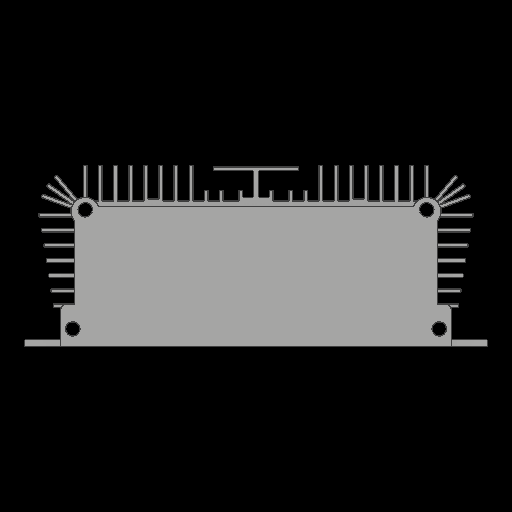
# Autodesk Inventor part: Daygreen-A2D12C100-Converter
Saved by Autodesk Inventor 2025.2 (Build 292293000, 293)
## iProperties
Created: 2025-11-13
Part Number: Daygreen-A2D12C100-Converter
Material: Generic
Document SubType Name: Modeling
Designer: valer
Density: 1 g/cm^3
Appearance: Default
Author: valer
Autodesk Inventor part; units mm, degrees
ref_plane "YZ Plane" through (0, 0, 0) normal (1, 0, 0) x (0, 1, 0)
ref_plane "XZ Plane" through (0, 0, 0) normal (0, 1, 0) x (-1, 0, 0)
sketch "Base" plane through (0, 0, 0) normal (0, 0, 1) x (1, 0, 0)
  line L0 (-65, -111.5) -> (65, -111.5)
  line L1 (65, -111.5) -> (65, 111.5)
  line L2 (65, 111.5) -> (-65, 111.5)
  line L3 (-65, 111.5) -> (-65, -111.5)
  line L4 (-65, -111.5) -> (65, 111.5) construction
  line L5 (65, -111.5) -> (-65, 111.5) construction
  line L6 (-91, 0) -> (91, 0) construction
  line L7 (0, -156.1) -> (0, 156.1) construction
  circle A0 centre (-59.5, 75.5) radius 2.5
  line L8 (-59.5, 78) -> (-65, 78)
  line L9 (-59.5, 73) -> (-65, 73)
  line L10 (-57, 75.5) -> (-65, 75.5) construction
  circle A1 centre (-59.5, 0) radius 2.5
  line L11 (-59.5, 2.5) -> (-65, 2.5)
  line L12 (-59.5, -2.5) -> (-65, -2.5)
  circle A2 centre (-59.5, -75.5) radius 2.5
  line L13 (-59.5, -78) -> (-65, -78)
  line L14 (-59.5, -73) -> (-65, -73)
  circle A3 centre (59.5, 75.5) radius 2.5
  line L15 (59.5, 78) -> (65, 78)
  line L16 (59.5, 73) -> (65, 73)
  circle A4 centre (59.5, 0) radius 2.5
  line L17 (59.5, 2.5) -> (65, 2.5)
  line L18 (59.5, -2.5) -> (65, -2.5)
  line L19 (59.5, -78) -> (65, -78)
  line L20 (59.5, -73) -> (65, -73)
  circle A5 centre (59.5, -75.5) radius 2.5
  point P0 (0, 0)
  dimension "d0" = 130
  dimension "d1" = 223
  dimension "d4" = 5
  dimension "d5" = 8
  dimension "d6" = 36
  constraints: 38 end point, 20 symmetric about line, 13 point on circle, 7 point on line, 6 centre point, 6 perpendicular, 4 tangent, 3 parallel, 2 midpoint, 1 equal radius, 1 horizontal, 4 other
  measures "d0" distance of L1.end L2.end
  measures "d1" distance of L0.end L1.end
  measures "d4" diameter of A0
  measures "d5" distance of L10.start L10.end
  measures "d6" distance between parallel lines of L10 L2
extrude "BaseFeature" add sketch "Base" along normal blind 2 contours L3 L13 A2 L14 L12 A1 L11 L9 A0 L8 L2 L1 L15 A3 L16 L17 A4 L18 L20 A5 L19 L0
sketch "BaseIndent" plane through (0, 0, 0) normal (0, 0, 1) x (1, 0, 0)
  line L0 (65, 111.5) -> (-65, 111.5) projected
  line L1 (-65, -111.5) -> (65, -111.5) projected
  line L2 (47.62, 111.5) -> (-47.62, 111.5)
  line L3 (-47.62, 111.5) -> (-47.62, -111.5)
  line L4 (-47.62, -111.5) -> (47.62, -111.5)
  line L5 (47.62, -111.5) -> (47.62, 111.5)
  line L6 (-65, 111.5) -> (-65, 78) projected
  line L7 (65, 78) -> (65, 111.5) projected
  point P0 (0, 0)
  point P1 (47.62, -111.5)
  point P2 (-47.62, 111.5)
  dimension "d7" = 17.38
  dimension "d8" = 17.38
  constraints: 8 end point, 2 parallel, 2 point on line, 1 horizontal, 1 perpendicular
  measures "d7" distance between parallel lines of L6 L3
  measures "d8" distance between parallel lines of L7 L5
extrude "BaseIndentFeature" cut sketch "BaseIndent" along normal blind 0.5
sketch "Wall" plane through (-65, -111.5, 2) normal (0, -1, 0) x (1, 0, 0)
  line L0 (0, -2) -> (17.38, -2) projected
  line L1 (10, -2) -> (120, -2)
  line L2 (120, -2) -> (120, 10)
  line L3 (120, 10) -> (10, 10)
  line L4 (10, 10) -> (10, -2)
  line L5 (14, 10) -> (116, 10)
  line L6 (116, 10) -> (116, 37.5)
  line L7 (116, 37.5) -> (14, 37.5)
  line L8 (14, 37.5) -> (14, 10)
  circle A0 centre (17, 36) radius 4
  line L9 (65, -10.5958) -> (65, 49.5748) construction
  line L10 (0, -2) -> (0, 0) projected
  circle A1 centre (113, 36) radius 4
  circle A2 centre (13.5, 3) radius 2
  line L11 (0, 0) -> (130, 0) projected
  circle A3 centre (17, 36.5) radius 2
  circle A4 centre (116.5, 3) radius 2
  circle A5 centre (113, 36.5) radius 2
  point P0 (65, -2)
  point P1 (65, 37.5)
  point P2 (65, 10)
  point P3 (20.7081, 37.5)
  point P4 (14, 33.3542)
  point P5 (116, 10)
  point P6 (116, 33.3542)
  point P7 (109.2919, 37.5)
  dimension "d11" = 12
  dimension "d12" = 39.5
  dimension "d13" = 102
  dimension "d14" = 10
  dimension "d18" = 8
  dimension "d19" = 48
  dimension "d20" = 1.5
  dimension "d21" = 4
  dimension "d24" = 3.5
  dimension "d25" = 5
  dimension "d27" = 3
  dimension "d28" = 1
  dimension "d61" = 4
  constraints: 16 end point, 6 centre point, 4 parallel, 3 midpoint, 3 point on line, 3 symmetric about line, 2 horizontal, 2 perpendicular, 3 other
  measures "d11" distance between parallel lines of L0 L3
  measures "d12" distance between parallel lines of L0 L7
  measures "d13" distance of L7.end L6.end
  measures "d14" distance between parallel lines of L10 L4
  measures "d18" diameter of A0
  measures "d19" distance from line of L9 A0.centre
  measures "d20" distance from line of L7 A0.centre
  measures "d21" diameter of A2
  measures "d24" distance from line of L4 A2.centre
  measures "d25" distance from line of L0 A2.centre
  measures "d27" distance from line of L8 A3.centre
  measures "d28" distance from line of L7 A3.centre
  measures "d61" diameter of A5
extrude "WallFeature" add sketch "Wall" along normal blind 1.6 contours L4 L11 L2 L1 L0 | L4 L3 L2 L11 | L8 A0 L7 A1 L6 L3 | A0 L7 A3 L8 | L8 L7 A3 A0 | A1 L7 A5 L6 | L6 L7 A5 A1
mirror "WallMirrorFeature" about plane through (0, 0, 0) normal (0, 1, 0) of "WallFeature"
fillet "WallFilletsFeature" radius 2 4 edges at (-55, -112.3, 12) (55, -112.3, 12) (-55, 112.3, 12) (55, 112.3, 12)
sketch "Heatsink" plane through (-65, -111.5, 2) normal (0, 1, 0) x (1, 0, 0)
  arc A0 (14, -33.3542) -> (20.7081, -37.5) centre (17, -36) ccw projected
  line L0 (19.6458, -39) -> (20.75, -39)
  line L1 (20.75, -39) -> (20.75, -49)
  line L2 (20.75, -49) -> (21.75, -49)
  line L3 (21.75, -49) -> (21.75, -39)
  line L4 (21.75, -39) -> (25, -39)
  line L5 (25, -39) -> (25, -49)
  line L6 (25, -49) -> (26, -49)
  line L7 (26, -49) -> (26, -39)
  line L8 (26, -39) -> (29.25, -39)
  line L9 (29.25, -39) -> (29.25, -49)
  line L10 (29.25, -49) -> (30.25, -49)
  line L11 (30.25, -49) -> (30.25, -39)
  line L12 (30.25, -39) -> (33.5, -39)
  line L13 (33.5, -39) -> (33.5, -49)
  line L14 (33.5, -49) -> (34.5, -49)
  line L15 (34.5, -49) -> (34.5, -39.5)
  line L16 (34.5, -39.5) -> (37.75, -39.5)
  line L17 (37.75, -39.5) -> (37.75, -49)
  line L18 (37.75, -49) -> (38.75, -49)
  line L19 (38.75, -49) -> (38.75, -39)
  line L20 (38.75, -39) -> (42, -39)
  line L21 (42, -39) -> (42, -49)
  line L22 (42, -49) -> (43, -49)
  line L23 (43, -49) -> (43, -39)
  line L24 (43, -39) -> (46.25, -39)
  line L25 (46.25, -39) -> (46.25, -49)
  line L26 (46.25, -49) -> (47.25, -49)
  line L27 (47.25, -49) -> (47.25, -39)
  line L28 (47.25, -39) -> (50.5, -39)
  line L29 (50.5, -39) -> (50.5, -42)
  line L30 (50.5, -42) -> (51.5, -42)
  line L31 (51.5, -42) -> (51.5, -39)
  line L32 (51.5, -39) -> (54.75, -39)
  line L33 (54.75, -39) -> (54.75, -42)
  line L34 (54.75, -42) -> (55.75, -42)
  line L35 (55.75, -42) -> (55.75, -39)
  line L36 (55.75, -39) -> (60.25, -39)
  line L37 (60.25, -39) -> (60.25, -42)
  line L38 (60.25, -42) -> (61.25, -42)
  line L39 (61.25, -42) -> (61.25, -40)
  line L40 (61.25, -40) -> (64.25, -40)
  line L41 (64.25, -40) -> (64.25, -47.5)
  line L42 (64.25, -47.5) -> (53, -47.5)
  line L43 (53, -47.5) -> (53, -48.5)
  line L44 (53, -48.5) -> (65, -48.5)
  line L45 (65, -48.5) -> (65, -37.5)
  line L46 (109.2919, -37.5) -> (20.7081, -37.5) projected
  line L47 (20.75, -39) -> (19.6458, -39)
  line L48 (17.5, -49) -> (17.5, -39.9686)
  line L49 (17.5, -49) -> (16.5, -49)
  line L50 (16.5, -49) -> (16.5, -39.9686)
  line L51 (14.832, -39.3615) -> (9.0268, -46.28)
  line L52 (9.0268, -46.28) -> (8.2607, -45.6372)
  line L53 (8.2607, -45.6372) -> (14.066, -38.7188)
  line L54 (14.0359, -38.6859) -> (6.6378, -43.8661)
  line L55 (6.6378, -43.8661) -> (6.0642, -43.0469)
  line L56 (6.0642, -43.0469) -> (13.4623, -37.8667)
  line L57 (13.0997, -36.8875) -> (4.613, -39.9764)
  line L58 (4.613, -39.9764) -> (4.955, -40.9161)
  line L59 (4.955, -40.9161) -> (13.4417, -37.8272)
  line L60 (4.0385, -35.5) -> (13.0314, -35.5)
  line L61 (4.0385, -35.5) -> (4.0385, -34.5)
  line L62 (4.0385, -34.5) -> (13.2919, -34.5)
  line L63 (14, -33.3542) -> (14, -10) projected
  line L64 (14, -31.25) -> (4.712, -31.25)
  line L65 (4.712, -31.25) -> (4.712, -30.25)
  line L66 (4.712, -30.25) -> (14, -30.25)
  line L67 (14, -27) -> (5.3854, -27)
  line L68 (5.3854, -27) -> (5.3854, -26)
  line L69 (5.3854, -26) -> (14, -26)
  line L70 (14, -22.75) -> (6.0589, -22.75)
  line L71 (6.0589, -22.75) -> (6.0589, -21.75)
  line L72 (6.0589, -21.75) -> (14, -21.75)
  line L73 (14, -18.5) -> (6.7323, -18.5)
  line L74 (6.7323, -18.5) -> (6.7323, -17.5)
  line L75 (6.7323, -17.5) -> (14, -17.5)
  line L76 (14, -14.25) -> (7.4058, -14.25)
  line L77 (7.4058, -14.25) -> (7.4058, -13.25)
  line L78 (7.4058, -13.25) -> (14, -13.25)
  line L79 (14, -10) -> (8, -10)
  line L80 (8, -10) -> (8, -9)
  line L81 (8, -9) -> (10.2679, -9)
  arc A1 (10, -8) -> (12, -10) centre (12, -8) ccw projected
  line L82 (6.351, -43.4565) -> (17, -36) construction
  line L83 (4.784, -40.4463) -> (17, -36) construction
  line L84 (8.6438, -45.9586) -> (17, -36) construction
  circle A2 centre (17, -36) radius 13 construction
  line L85 (4.0385, -35) -> (8, -10) construction
  line L86 (10, -8) -> (10, 2) projected
  line L87 (65, 12.2) -> (65, -59.2) construction
  line L88 (65, -37.5) -> (65, 2)
  line L89 (10, 2) -> (120, 2) projected
  line L90 (14, -10) -> (12, -10) projected
  arc A3 (118, -10) -> (120, -8) centre (118, -8) ccw projected
  line L91 (118, -10) -> (116, -10) projected
  line L92 (116, -10) -> (116, -33.3542) projected
  arc A4 (109.2919, -37.5) -> (116, -33.3542) centre (113, -36) ccw projected
  line L93 (109.2919, -37.5) -> (20.7081, -37.5) projected
  arc A5 (14, -33.3542) -> (20.7081, -37.5) centre (17, -36) ccw projected
  line L94 (14, -33.3542) -> (14, -10) projected
  line L95 (14, -10) -> (12, -10) projected
  arc A6 (10, -8) -> (12, -10) centre (12, -8) ccw projected
  line L96 (10, -8) -> (10, 2) projected
  line L97 (10, 2) -> (120, 2) projected
  line L98 (120, 2) -> (120, -8) projected
  circle A7 centre (17, -36.5) radius 2 projected
  circle A8 centre (116.5, -3) radius 2 projected
  circle A9 centre (13.5, -3) radius 2 projected
  circle A10 centre (113, -36.5) radius 2 projected
  point P0 (48.875, -39)
  point P1 (51, -42)
  point P2 (7.4058, -13.75)
  point P3 (6.7323, -18)
  point P4 (6.0589, -22.25)
  point P5 (5.3854, -26.5)
  point P6 (4.712, -30.75)
  dimension "d30" = 12
  dimension "d31" = 11
  dimension "d32" = 1
  dimension "d33" = 1.5
  dimension "d34" = 3.25
  dimension "d35" = 2
  dimension "d36" = 2.5
  dimension "d37" = 10
  dimension "d38" = 3
  dimension "d39" = 4.5
  dimension "d40" = 0.75
  dimension "d41" = 125
  dimension "d42" = 15
  dimension "d43" = 15
  dimension "d44" = 3.25
  dimension "d45" = 3.25
  dimension "d46" = 3.25
  dimension "d47" = 3.25
  dimension "d48" = 3.25
  dimension "d49" = 3.25
  dimension "d50" = 20
  dimension "d51" = 40
  dimension "d52" = 2
  dimension "d53" = 3.25
  dimension "d54" = 3
  constraints: 170 end point, 45 perpendicular, 29 equal length, 17 collinear, 14 horizontal, 12 midpoint, 9 point on line, 8 parallel, 5 point on circle, 1 centre point, 1 coincident, 1 vertical, 23 other
  measures "d30" distance of L43.end L44.end
  measures "d31" distance of L44.end L45.end
  measures "d32" distance between parallel lines of L3 L1
  measures "d33" distance between parallel lines of L46 L4
  measures "d34" distance between parallel lines of L5 L3
  measures "d35" distance between parallel lines of L46 L16
  measures "d36" distance between parallel lines of L46 L40
  measures "d37" distance of L0.end L1.end
  measures "d38" vertical distance of point (48.875, -39) point (51, -42)
  measures "d39" distance of L35.end L36.end
  measures "d40" distance between parallel lines of L45 L41
  measures "d42" angle of L53 L54
  measures "d43" angle of L59 L56
  measures "d44" distance between parallel lines of L79 L78
  measures "d45" distance between parallel lines of L76 L75
  measures "d46" distance between parallel lines of L73 L72
  measures "d47" distance between parallel lines of L70 L69
  measures "d48" distance between parallel lines of L67 L66
  measures "d49" distance between parallel lines of L64 L62
  measures "d50" angle of L60 L57
  measures "d51" angle of L50 L51
  measures "d52" distance from line of L86 L80.end
  measures "d53" distance between parallel lines of L48 L1
  measures "d54" distance of L39.end L40.end
extrude "HeatSinkFeature" add sketch "Heatsink" along normal up to surface (223 mm away) contours L63 L79 A1 L86 L89 L88 L46 A0 | A0 L60 L61 L62 | L64 L65 L66 L63 | A0 L59 L58 L57 | L67 L68 L69 L63 | A0 L54 L55 L56 | L70 L71 L72 L63 | A0 L51 L52 L53 | L73 L74 L75 L63 | A0 L48 L49 L50 | L76 L77 L78 L63 | A0 L46 L45 L44 L43 L42 L41 L40 L39 L38 L37 L36 L35 L34 L33 L32 L31 L30 L29 L28 L27 L26 L25 L24 L23 L22 L21 L20 L19 L18 L17 L16 L15 L14 L13 L12 L11 L10 L9 L8 L7 L6 L5 L4 L3 L2 L1 L0 | L79 L80 L81 A1
mirror "HeatSinkMirrorFeature" about plane through (0, 0, 0) normal (1, 0, 0) of "HeatSinkFeature"
sketch "Terminal" plane through (-55, 113.1, 0) normal (0, 1, 0) x (1, 0, 0)
  line L0 (94.25, -26) -> (15.75, -26)
  line L1 (15.75, -26) -> (15.75, -13)
  line L2 (15.75, -13) -> (94.25, -13)
  line L3 (94.25, -13) -> (94.25, -26)
  line L4 (55, 10.2) -> (55, -61.2) construction
  line L5 (99.2919, -39.5) -> (10.7081, -39.5) projected
  line L6 (55, -39.5) -> (55, 0) construction
  line L7 (0, 0) -> (110, 0) projected
  point P0 (55, 0)
  point P1 (55, -26)
  dimension "d57" = 78.5
  dimension "d58" = 13
  dimension "d59" = 13
  dimension "d60" = 13.5
  constraints: 10 end point, 3 midpoint, 2 parallel, 2 point on line, 1 horizontal, 1 perpendicular
  measures "d57" distance of L0.start L0.end
  measures "d58" distance of L2.end L0.start
  measures "d59" distance between parallel lines of L7 L2
  measures "d60" distance between parallel lines of L5 L0
extrude "TerminalFeature" add sketch "Terminal" along normal blind 11.7
sketch "TerminalCells" plane through (-39.25, 113.1, 26) normal (0, 0, 1) x (1, 0, 0)
  line L0 (78.5, 11.7) -> (0, 11.7) projected
  line L1 (2.5, 11.7) -> (14.2, 11.7)
  line L2 (14.2, 11.7) -> (14.2, 0)
  line L3 (14.2, 0) -> (2.5, 0)
  line L4 (2.5, 0) -> (2.5, 11.7)
  line L5 (16.7, 11.7) -> (28.4, 11.7)
  line L6 (28.4, 11.7) -> (28.4, 0)
  line L7 (28.4, 0) -> (16.7, 0)
  line L8 (16.7, 0) -> (16.7, 11.7)
  line L9 (76, 11.7) -> (64.3, 11.7)
  line L10 (64.3, 11.7) -> (64.3, 0)
  line L11 (64.3, 0) -> (76, 0)
  line L12 (76, 0) -> (76, 11.7)
  line L13 (61.8, 11.7) -> (53.5, 11.7)
  line L14 (53.5, 11.7) -> (53.5, 0)
  line L15 (53.5, 0) -> (61.8, 0)
  line L16 (61.8, 0) -> (61.8, 11.7)
  line L17 (51, 11.7) -> (39.3, 11.7)
  line L18 (39.3, 11.7) -> (39.3, 0)
  line L19 (39.3, 0) -> (51, 0)
  line L20 (51, 0) -> (51, 11.7)
  line L21 (83.5419, 0) -> (-5.0419, 0) projected
  line L22 (0, 0) -> (0, 11.7) projected
  line L23 (78.5, 0) -> (78.5, 11.7) projected
  point P0 (39.25, -113.1)
  point P1 (51, 11.7)
  point P2 (39.3, 11.7)
  dimension "d64" = 11.7
  dimension "d65" = 2.5
  dimension "d66" = 2.5
  dimension "d67" = 2.5
  dimension "d68" = 2.5
  dimension "d69" = 2.5
  dimension "d70" = 8.3
  constraints: 40 end point, 10 parallel, 8 point on line, 5 collinear, 5 horizontal, 5 perpendicular
  measures "d64" distance between parallel lines of L12 L10
  measures "d65" distance between parallel lines of L4 L22
  measures "d66" distance between parallel lines of L8 L2
  measures "d67" distance between parallel lines of L23 L12
  measures "d68" distance between parallel lines of L16 L10
  measures "d69" distance between parallel lines of L14 L20
  measures "d70" distance between parallel lines of L16 L14
extrude "TerminalCellsFeature" cut sketch "TerminalCells" against normal blind 6 contours L12 L11 L10 L0 | L16 L15 L14 L0 | L20 L19 L18 L0 | L6 L7 L8 L0 | L2 L3 L4 L0
sketch "TerminalBreak" plane through (-10.85, 113.1, 26) normal (0, 0, 1) x (1, 0, 0)
  line L0 (10.9, 0) -> (10.9, 11.7) projected
  line L1 (0, 11.7) -> (10.9, 11.7) projected
  line L2 (0, 11.7) -> (0, 0) projected
  line L3 (10.9, 0) -> (0, 0) projected
  line L4 (2.5, 0) -> (2.5, 11.7)
  line L5 (8.4, 0) -> (8.4, 11.7)
  point P0 (10.85, -113.1)
  dimension "d73" = 2.5
  dimension "d74" = 2.5
  constraints: 4 end point, 4 point on line, 2 perpendicular
  measures "d73" distance between parallel lines of L2 L4
  measures "d74" distance between parallel lines of L0 L5
extrude "TerminalBreakFeature" cut sketch "TerminalBreak" against normal through all contours L3 L4 L1 L5
sketch "TerminalChannels" plane through (-55, 124.8, 0) normal (0, 1, 0) x (1, 0, 0)
  line L0 (46.65, -26) -> (46.65, -13) projected
  line L1 (46.65, -13) -> (15.75, -13) projected
  line L2 (15.75, -13) -> (15.75, -26) projected
  line L3 (15.75, -26) -> (18.25, -26) projected
  line L4 (18.25, -26) -> (18.25, -20) projected
  line L5 (18.25, -20) -> (29.95, -20) projected
  line L6 (29.95, -20) -> (29.95, -26) projected
  line L7 (29.95, -26) -> (32.45, -26) projected
  line L8 (32.45, -26) -> (32.45, -20) projected
  line L9 (32.45, -20) -> (44.15, -20) projected
  line L10 (44.15, -20) -> (44.15, -26) projected
  line L11 (44.15, -26) -> (46.65, -26) projected
  line L12 (52.55, -13) -> (52.55, -26) projected
  line L13 (52.55, -26) -> (55.05, -26) projected
  line L14 (55.05, -26) -> (55.05, -20) projected
  line L15 (55.05, -20) -> (66.75, -20) projected
  line L16 (66.75, -20) -> (66.75, -26) projected
  line L17 (66.75, -26) -> (69.25, -26) projected
  line L18 (69.25, -26) -> (69.25, -20) projected
  line L19 (69.25, -20) -> (77.55, -20) projected
  line L20 (77.55, -20) -> (77.55, -26) projected
  line L21 (77.55, -26) -> (80.05, -26) projected
  line L22 (80.05, -26) -> (80.05, -20) projected
  line L23 (80.05, -20) -> (91.75, -20) projected
  line L24 (91.75, -20) -> (91.75, -26) projected
  line L25 (91.75, -26) -> (94.25, -26) projected
  line L26 (94.25, -26) -> (94.25, -13) projected
  line L27 (94.25, -13) -> (52.55, -13) projected
  line L28 (31.2, -26) -> (31.2, -13)
  line L29 (29.95, -20) -> (18.25, -20) projected
  line L30 (28.35, -20) -> (28.1, -15)
  line L31 (28.1, -15) -> (20.1, -15)
  line L32 (20.1, -15) -> (19.85, -20)
  line L33 (24.1, -15) -> (24.1, -20) construction
  line L34 (34.05, -20) -> (34.3, -15)
  line L35 (34.3, -15) -> (42.3, -15)
  line L36 (42.3, -15) -> (42.55, -20)
  line L37 (73.4, -20) -> (73.4, -13) construction
  line L38 (65.15, -20) -> (64.9, -15)
  line L39 (64.9, -15) -> (56.9, -15)
  line L40 (56.9, -15) -> (56.65, -20)
  line L41 (66.75, -20) -> (55.05, -20) projected
  line L42 (60.9, -20) -> (60.9, -15) construction
  line L43 (81.65, -20) -> (81.9, -15)
  line L44 (81.9, -15) -> (89.9, -15)
  line L45 (89.9, -15) -> (90.15, -20)
  point P0 (55, 0)
  point P1 (19.85, -20)
  point P2 (42.55, -20)
  dimension "d77" = 8.5
  dimension "d78" = 8
  dimension "d79" = 2
  dimension "d80" = 8.5
  constraints: 32 end point, 8 midpoint, 8 symmetric about line, 4 point on line, 3 equal length, 2 perpendicular, 1 collinear, 1 horizontal, 1 parallel
  measures "d77" distance of L32.end L30.start
  measures "d78" distance of L30.end L31.end
  measures "d79" distance between parallel lines of L1 L31
  measures "d80" distance of L40.end L38.start
extrude "TerminalChannelsFeature" cut sketch "TerminalChannels" against normal up to surface (11.7 mm away) contours L9 L34 L35 L36 | L5 L32 L31 L30 | L40 L39 L38 L15 | L23 L43 L44 L45
ref_plane "TerminalPlatePlane" through (-55, 125.05, 0) normal (0, 1, 0) x (1, 0, 0)
sketch "TerminalPlates" plane through (-55, 125.05, 0) normal (0, 1, 0) x (1, 0, 0)
  line L0 (29.95, -26) -> (29.95, -20) projected
  line L1 (18.25, -26) -> (18.25, -20) projected
  line L2 (29.95, -20) -> (18.25, -20)
  line L3 (18.25, -20) -> (18.25, -21)
  line L4 (18.25, -21) -> (29.95, -21)
  line L5 (29.95, -21) -> (29.95, -20)
  line L6 (44.15, -26) -> (44.15, -20) projected
  line L7 (32.45, -26) -> (32.45, -20) projected
  line L8 (44.15, -20) -> (32.45, -20)
  line L9 (32.45, -20) -> (32.45, -21)
  line L10 (32.45, -21) -> (44.15, -21)
  line L11 (44.15, -21) -> (44.15, -20)
  line L12 (66.75, -26) -> (66.75, -20) projected
  line L13 (55.05, -26) -> (55.05, -20) projected
  line L14 (66.75, -20) -> (55.05, -20)
  line L15 (55.05, -20) -> (55.05, -21)
  line L16 (55.05, -21) -> (66.75, -21)
  line L17 (66.75, -21) -> (66.75, -20)
  line L18 (91.75, -26) -> (91.75, -20) projected
  line L19 (80.05, -26) -> (80.05, -20) projected
  line L20 (91.75, -20) -> (80.05, -20)
  line L21 (80.05, -20) -> (80.05, -21)
  line L22 (80.05, -21) -> (91.75, -21)
  line L23 (91.75, -21) -> (91.75, -20)
  point P0 (55, 0)
  point P1 (18.25, -20)
  point P2 (29.95, -21)
  point P3 (32.45, -20)
  point P4 (91.75, -21)
  dimension "d84" = 1
  constraints: 32 end point, 8 parallel, 4 horizontal, 4 perpendicular, 4 point on line, 3 collinear
  measures "d84" distance from line of L1.end L4
extrude "TerminalPlatesFeature" add sketch "TerminalPlates" against normal up to surface (11.95 mm away)
sketch "TerminalBoltRings" plane through (-36.75, 125.05, 21) normal (0, 0, 1) x (1, 0, 0)
  line L0 (11.7, -11.95) -> (0, -11.95) projected
  line L1 (11.7, -0.25) -> (11.7, -11.95) projected
  line L2 (11.7, 0) -> (11.7, -0.25) projected
  line L3 (0, 0) -> (11.7, 0) projected
  line L4 (0, 0) -> (0, -0.25) projected
  line L5 (0, -11.95) -> (0, -0.25) projected
  line L6 (25.9, -11.95) -> (14.2, -11.95) projected
  line L7 (25.9, -0.25) -> (25.9, -11.95) projected
  line L8 (25.9, 0) -> (25.9, -0.25) projected
  line L9 (14.2, 0) -> (25.9, 0) projected
  line L10 (14.2, 0) -> (14.2, -0.25) projected
  line L11 (14.2, -11.95) -> (14.2, -0.25) projected
  line L12 (48.5, -11.95) -> (36.8, -11.95) projected
  line L13 (48.5, -0.25) -> (48.5, -11.95) projected
  line L14 (48.5, 0) -> (48.5, -0.25) projected
  line L15 (36.8, 0) -> (48.5, 0) projected
  line L16 (36.8, 0) -> (36.8, -0.25) projected
  line L17 (36.8, -11.95) -> (36.8, -0.25) projected
  line L18 (73.5, -11.95) -> (61.8, -11.95) projected
  line L19 (73.5, -0.25) -> (73.5, -11.95) projected
  line L20 (73.5, 0) -> (73.5, -0.25) projected
  line L21 (61.8, 0) -> (73.5, 0) projected
  line L22 (61.8, 0) -> (61.8, -0.25) projected
  line L23 (61.8, -11.95) -> (61.8, -0.25) projected
  line L24 (11.7, -11.95) -> (0, -0.25) construction
  circle A0 centre (5.85, -6.1) radius 4
  line L25 (11.7, -0.25) -> (14.2, -0.25) projected
  line L26 (25.9, -11.95) -> (14.2, -0.25) construction
  circle A1 centre (20.05, -6.1) radius 4
  line L27 (34.3, -0.25) -> (36.8, -0.25) projected
  line L28 (48.5, -11.95) -> (36.8, -0.25) construction
  circle A2 centre (42.65, -6.1) radius 4
  line L29 (59.3, -0.25) -> (61.8, -0.25) projected
  line L30 (73.5, -11.95) -> (61.8, -0.25) construction
  circle A3 centre (67.65, -6.1) radius 4
  point P0 (36.75, -125.05)
  dimension "d87" = 8
  constraints: 8 end point, 4 centre point, 4 midpoint, 3 equal radius
  measures "d87" diameter of A0
extrude "TerminalBoltRingsFeature" add sketch "TerminalBoltRings" along normal blind 1 contours A0 | A1 | A2 | A3
sketch "TerminalBoltBodies" plane through (30.9, 118.95, 22) normal (0, 0, 1) x (1, 0, 0)
  circle A0 centre (-47.6, 0) radius 4 projected
  circle A1 centre (-61.8, 0) radius 4 projected
  circle A2 centre (-25, 0) radius 4 projected
  circle A3 centre (0, 0) radius 4 projected
  circle A4 centre (-61.8, 0) radius 2
  circle A5 centre (-47.6, 0) radius 2
  circle A6 centre (-25, 0) radius 2
  circle A7 centre (0, 0) radius 2
  point P0 (-30.9, -118.95)
  dimension "d90" = 4
  constraints: 4 centre point, 4 coincident, 3 equal radius
  measures "d90" diameter of A4
extrude "TerminalBoltBodiesFeature" add sketch "TerminalBoltBodies" along normal blind 3 contours A4 | A5 | A6 | A7
sketch "TerminalBoltHeads" plane through (30.9, 118.95, 25) normal (0, 0, 1) x (1, 0, 0)
  circle A0 centre (0, 0) radius 2 projected
  circle A1 centre (-25, 0) radius 2 projected
  circle A2 centre (-47.6, 0) radius 2 projected
  circle A3 centre (-61.8, 0) radius 2 projected
  circle A4 centre (0, 0) radius 4 projected
  circle A5 centre (0, 0) radius 4
  circle A6 centre (-25, 0) radius 4 projected
  circle A7 centre (-47.6, 0) radius 4 projected
  circle A8 centre (-61.8, 0) radius 4 projected
  point P0 (-30.9, -118.95)
  dimension "d93" = 8
  constraints: 1 centre point, 1 coincident
  measures "d93" diameter of A5
extrude "TerminalBoltHeadsFeature" add sketch "TerminalBoltHeads" along normal blind 3 contours A0 | A1 | A2 | A3 | A4 | A6 | A7 | A8
fillet "TerminalBoltFilletsFeature" radius 3 4 edges at (26.9, 118.95, 28) (1.9, 118.95, 28) (-20.7, 118.95, 28) (-34.9, 118.95, 28)
sketch "TerminalAccPlate" plane through (25.05, 125.05, 21) normal (0, 0, 1) x (1, 0, 0)
  circle A0 centre (5.85, -6.1) radius 4 projected
  line L0 (11.7, -11.95) -> (0, -11.95) projected
  line L1 (11.7, -0.25) -> (11.7, -11.95) projected
  line L2 (11.7, 0) -> (11.7, -0.25) projected
  line L3 (0, 0) -> (11.7, 0) projected
  line L4 (0, 0) -> (0, -0.25) projected
  line L5 (0, -11.95) -> (0, -0.25) projected
  line L6 (9.6, -12.244) -> (2.1, -12.244)
  line L7 (2.1, -12.244) -> (2.1, 2.5)
  line L8 (2.1, 2.5) -> (9.6, 2.5)
  line L9 (9.6, 2.5) -> (9.6, -12.244)
  line L10 (-2.9, -11.95) -> (-10.4, -11.95)
  line L11 (-10.4, -11.95) -> (-10.4, 2.5)
  line L12 (-10.4, 2.5) -> (-2.9, 2.5)
  line L13 (-2.9, 2.5) -> (-2.9, -11.95)
  line L14 (-2.5, -11.95) -> (-10.8, -11.95) projected
  line L15 (2.1, 2.5) -> (-2.9, 2.5)
  line L16 (9.6, 2.5) -> (9.6, 3)
  line L17 (9.6, 3) -> (-10.4, 3)
  line L18 (-10.4, 3) -> (-10.4, 2.5)
  point P0 (-25.05, -125.05)
  point P1 (-6.65, -11.95)
  point P2 (9.6, -4.7081)
  point P3 (2.1, -4.7081)
  point P4 (2.1, -7.4919)
  point P5 (2.1, -11.95)
  point P6 (9.6, -11.95)
  point P7 (9.6, -7.4919)
  dimension "d97" = 0.5
  dimension "d98" = 7.5
  dimension "d99" = 7.5
  dimension "d100" = 2.1
  dimension "d101" = 2.1
  dimension "d102" = 3
  constraints: 24 end point, 4 parallel, 4 perpendicular, 3 collinear, 2 horizontal, 2 midpoint, 1 vertical
  measures "d97" distance between parallel lines of L17 L15
  measures "d98" distance between parallel lines of L11 L13
  measures "d99" distance between parallel lines of L7 L9
  measures "d100" distance between parallel lines of L9 L1
  measures "d101" distance between parallel lines of L5 L7
  measures "d102" distance between parallel lines of L17 L3
extrude "TerminalAccPlateFeature" add sketch "TerminalAccPlate" along normal blind 0.5 contours A0 L9 | L9 A0 L7 | A0 L7 L3 L9 | L9 L0 L7 A0 | L7 A0 | L3 L7 L8 L9 | L8 L15 L12 L18 L17 L16 | L13 L10 L11 L12
sketch "TerminalAccPlateBend" plane through (34.65, 125.05, 21) normal (1, 0, 0) x (0, 0, -1)
  line L0 (0, 3) -> (6.5, 3)
  line L1 (6.5, 3) -> (6.5, 2.5)
  line L2 (6.5, 2.5) -> (0, 2.5)
  line L3 (0, 2.5) -> (0, 3)
  point P0 (21, -125.05)
  dimension "d105" = 6.5
  dimension "d106" = 0.5
  constraints: 8 end point, 2 parallel, 1 horizontal, 1 perpendicular
  measures "d105" distance of L0.start L0.end
  measures "d106" distance between parallel lines of L0 L2
extrude "TerminalAccPlateBendFeature" add sketch "TerminalAccPlateBend" against normal up to surface (20 mm away)
fillet "TerminalAccPlateBendFilletFeature" radius 0.5 1 edges at (24.65, 128.05, 21.5)
fillet "TerminalAccPlateFilletsFeature" radius 2 2 edges at (34.65, 127.8, 14.5) (14.65, 127.8, 14.5)
sketch "TerminalAccSubplate" plane through (25.05, 125.05, 21.5) normal (0, 0, 1) x (1, 0, 0)
  line L0 (-10.4, 2.5) -> (-2.9, 2.5) projected
  line L1 (-10.4, 2.5) -> (-10.4, -11.95) projected
  line L2 (-2.9, -11.95) -> (-10.4, -11.95) projected
  line L3 (-2.9, -11.95) -> (-2.9, 2.5) projected
  line L4 (-2.9, -1.95) -> (-10.4, -1.95)
  point P0 (-25.05, -125.05)
  dimension "d111" = 10
  constraints: 2 end point, 2 point on line, 1 perpendicular
  measures "d111" distance between parallel lines of L4 L2
extrude "TerminalAccSubplateFeature" add sketch "TerminalAccSubplate" along normal blind 1 contours L4 L3 L2 L1
sketch "TerminalAccBolt" plane through (25.05, 125.05, 22.5) normal (0, 0, 1) x (1, 0, 0)
  line L0 (-2.9, -11.95) -> (-2.9, -1.95) projected
  line L1 (-2.9, -1.95) -> (-10.4, -1.95) projected
  line L2 (-10.4, -1.95) -> (-10.4, -11.95) projected
  line L3 (-2.9, -11.95) -> (-10.4, -11.95) projected
  line L4 (-10.4, -11.95) -> (-2.9, -1.95) construction
  circle A0 centre (-6.65, -6.95) radius 3
  point P0 (-25.05, -125.05)
  dimension "d114" = 6
  constraints: 2 end point, 1 centre point, 1 midpoint
  measures "d114" diameter of A0
extrude "TerminalAccBoltFeature" add sketch "TerminalAccBolt" along normal blind 3 contours A0
fillet "TerminalAccBoltFilletFeature" radius 2.5 1 edges at (15.4, 118.1, 25.5)
equation "\"d8\" = d7"
equation "\"d44\" = d34"
equation "\"d45\" = d34"
equation "\"d46\" = d34"
equation "\"d47\" = d34"
equation "\"d48\" = d34"
equation "\"d49\" = d34"
equation "\"d53\" = d34"
body "Solid1"
